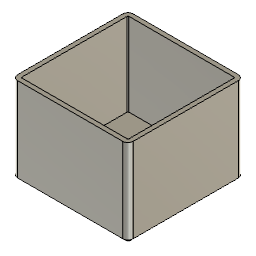
Insert (Autodesk Fusion 360 design; units mm, degrees)
part number: 2025-07-14-16-32-23-053
Autodesk Fusion 360 part; units mm, degrees
note: some values were not read from the file. Chosen so that the rebuilt part matches the saved one: that a step has no effect.
sketch "Sketch1" plane through (0, 0, 0) normal (0, 0, 1) x (1, 0, 0)
  line L0 (1.8, 0) -> (37.8, 0)
  line L1 (39.6, 1.8) -> (39.6, 37.8)
  line L2 (37.8, 39.6) -> (1.8, 39.6)
  line L3 (0, 37.8) -> (0, 1.8)
  arc A0 (39.6, 37.8) -> (37.8, 39.6) centre (37.8, 37.8) ccw
  arc A1 (1.8, 39.6) -> (0, 37.8) centre (1.8, 37.8) ccw
  arc A2 (0, 1.8) -> (1.8, 0) centre (1.8, 1.8) ccw
  arc A3 (37.8, 0) -> (39.6, 1.8) centre (37.8, 1.8) ccw
  point P0 (39.6, 0)
  point P1 (0, 39.6)
  dimension "d3" = 39.6
  dimension "d4" = 39.6
  dimension "d6" = 1.8
  dimension "d7" = 1.8
  dimension "d8" = 1.8
  dimension "d9" = 1.8
  constraint horizontal L0
  constraint vertical L1
  constraint horizontal L2
  constraint vertical L3
  constraint tangent L1 A0
  constraint tangent L2 A0
  constraint coincident P1 L2
  constraint coincident P1 L3
  constraint tangent L2 A1
  constraint tangent L3 A1
  constraint coincident origin L0
  constraint coincident origin L3
  constraint tangent L0 A2
  constraint tangent L3 A2
  constraint coincident P0 L0
  constraint coincident P0 L1
  constraint tangent L0 A3
  constraint tangent L1 A3
  measures "d3" distance of origin P0
  measures "d4" distance of origin P1
  measures "d6" radius of A0
  measures "d7" radius of A1
  measures "d8" radius of A2
  measures "d9" radius of A3
extrude "Extrude1" add sketch "Sketch1" along normal blind 29.9 makes body 1
shell "Shell1" thickness 1.5 removed faces 1 at (13.2, 13.8, 29.9) on bodies 1
sketch "Sketch5" plane through (0, 0, 1.5) normal (0, 0, 1) x (-1, 0, 0)
  line L0 (-0.75, -38.1) -> (-0.75, -1.5)
  line L1 (-1.8, -38.1) -> (-37.8, -38.1)
  line L2 (-37.8, -1.5) -> (-1.8, -1.5)
  line L3 (-1.5, -1.8) -> (-1.5, -37.8)
  line L4 (-1.8, -1.5) -> (-37.8, -1.5)
  line L5 (-38.1, -1.8) -> (-38.1, -37.8)
  line L6 (-37.8, -38.1) -> (-1.8, -38.1)
  line L7 (-1.5, -37.8) -> (-1.5, -1.8)
  arc A0 (-37.8, -1.5) -> (-38.1, -1.8) centre (-37.8, -1.8) ccw
  arc A1 (-38.1, -37.8) -> (-37.8, -38.1) centre (-37.8, -37.8) ccw
  arc A2 (-1.8, -38.1) -> (-1.5, -37.8) centre (-1.8, -37.8) ccw
  arc A3 (-1.5, -1.8) -> (-1.8, -1.5) centre (-1.8, -1.8) ccw
  dimension "d64" = 0.75
  constraint coincident L0.end L2
  constraint horizontal L0.start L1.start
  constraint vertical L0
  measures "d64" distance of origin L0
extrude "Extrude4" add sketch "Sketch5" along normal blind 28.4 thin wall 1.5 centred separate body open curves L0 makes body 2
pattern_linear "R-Pattern2" [no effect]
sketch "Sketch9" plane through (0, 0, 1.5) normal (0, 0, 1) x (-1, 0, 0)
  line L0 (-1.5, -0.75) -> (-38.1, -0.75)
  line L1 (-1.5, -1.8) -> (-1.5, -37.8)
  line L2 (-38.1, -37.8) -> (-38.1, -1.8)
  line L3 (-37.8, -1.5) -> (-1.8, -1.5)
  line L4 (-1.8, -1.5) -> (-37.8, -1.5)
  line L5 (-38.1, -1.8) -> (-38.1, -37.8)
  line L6 (-37.8, -38.1) -> (-1.8, -38.1)
  line L7 (-1.5, -37.8) -> (-1.5, -1.8)
  arc A0 (-37.8, -1.5) -> (-38.1, -1.8) centre (-37.8, -1.8) ccw
  arc A1 (-38.1, -37.8) -> (-37.8, -38.1) centre (-37.8, -37.8) ccw
  arc A2 (-1.8, -38.1) -> (-1.5, -37.8) centre (-1.8, -37.8) ccw
  arc A3 (-1.5, -1.8) -> (-1.8, -1.5) centre (-1.8, -1.8) ccw
  dimension "d65" = 0.75
  constraint coincident L0.start L1
  constraint coincident L0.end L2
  measures "d65" distance of origin L0
extrude "Extrude7" add sketch "Sketch9" along normal blind 28.4 thin wall 1.5 centred separate body open curves L0 makes body 3
pattern_linear "R-Pattern1" [no effect]
delete_body "RemoveBody1" bodies 2
delete_body "RemoveBody2" bodies 3
chamfer "Chamfer4" distance 1 angle 45 8 edges at (19.8, 0, 0) (39.0728, 0.5272, 0) (39.6, 19.8, 0) (39.0728, 39.0728, 0) (19.8, 39.6, 0) (0.5272, 39.0728, 0) (0, 19.8, 0) (0.5272, 0.5272, 0) on bodies 1
equation "Length = 40 mm"
equation "Width = 40 mm"
equation "d3 = Length - 0.4 mm"
equation "d4 = Width - 0.4 mm"
equation "CornerRadius = 1.8 mm"
equation "d6 = CornerRadius"
equation "d7 = CornerRadius"
equation "d8 = CornerRadius"
equation "d9 = CornerRadius"
equation "Height = 30 mm"
equation "d11 = Height - 0.1 mm"
equation "Columns = 1"
equation "Rows = 1"
equation "d34 = Height - 1.6 mm"
equation "LengthSectionDistance = ( Length - 1.5 mm ) / Columns"
equation "WidthSectionDistance = ( Width - 1.5 mm ) / Rows"
equation "d52 = Height - 1.6 mm"
equation "d54 = Rows"
equation "d56 = WidthSectionDistance"
equation "d58 = Columns"
equation "d60 = LengthSectionDistance"
